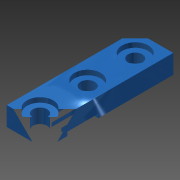
# Autodesk Inventor part: XCarriageBeltClamp
Saved by Autodesk Inventor 2015 (Build 190159000, 159)
## iProperties
Created: 2014-08-22
Part Number: XCarriageBeltClamp
Material: ABS Plastic
Document SubType Name: Modeling
Designer: t_clevj
Density: 1.06 g/cm^3
Appearance: Cyan
Author: t_clevj
Autodesk Inventor part; units mm, degrees
ref_plane "YZ Plane" through (0, 0, 0) normal (1, 0, 0) x (0, 1, 0)
ref_plane "XZ Plane" through (0, 0, 0) normal (0, 1, 0) x (-1, 0, 0)
ref_plane "XY Plane" through (0, 0, 0) normal (0, 0, 1) x (1, 0, 0)
sketch "Sketch1" plane through (0, 0, 0) normal (0, 0, 1) x (1, 0, 0)
  line L0 (0, 0) -> (8, 0)
  line L1 (8, 0) -> (8, 27)
  line L2 (8, 27) -> (0, 27)
  line L3 (0, 27) -> (0, 0)
  dimension "d0" = 27
  dimension "d1" = 8
  constraints: 8 end point, 2 parallel, 1 horizontal, 1 perpendicular
  measures "d0" distance of L2.end L0.start
  measures "d1" distance of L0.start L0.end
extrude "Extrusion1" add sketch "Sketch1" along normal blind 4
sketch "Sketch2" plane through (0, 0, 4) normal (0, 0, 1) x (1, 0, 0)
  line L0 (0, 0) -> (8, 0) projected
  line L1 (8, 0) -> (8, 27) projected
  point P0 (4, 23)
  point P1 (4, 13)
  point P2 (4, 3)
  dimension "d4" = 3
  dimension "d5" = 20
  dimension "d6" = 10
  dimension "d7" = 4
  constraints: 2 vertical alignment
  measures "d4" distance from line of L0 point (4, 3)
  measures "d5" distance of point (4, 23) point (4, 3)
  measures "d6" distance of point (4, 3) point (4, 13)
  measures "d7" distance from line of L1 point (4, 3)
hole "Hole1" at (4, 23, 4) at (4, 13, 4) at (4, 3, 4) direction (0, 0, -1) diameter 3 end up to face face through (2.6667, 18, 0) facing (0, 0, -1) counterbore diameter 5.5 counterbore depth 1
sketch "Sketch3" plane through (0, 0, 0) normal (0, 0, -1) x (-1, 0, 0)
  line L0 (-8, 0) -> (-8, 27) projected
  line L1 (-8, 21.25) -> (0, 21.25) construction
  line L2 (0, 27) -> (0, 0) construction
  line L3 (-8, 0) -> (-8, 27) construction
  line L4 (-8, 14.75) -> (0, 14.75) construction
  line L5 (-8, 21.25) -> (-6.7, 21.25)
  line L6 (-6.7, 21.25) -> (-6.7, 14.75)
  line L7 (-6.7, 14.75) -> (-8, 14.75)
  line L8 (-8, 14.75) -> (-8, 21.25)
  line L9 (-6, 21.25) -> (-4.7, 21.25)
  line L10 (-4.7, 21.25) -> (-4.7, 14.75)
  line L11 (-4.7, 14.75) -> (-6, 14.75)
  line L12 (-6, 14.75) -> (-6, 21.25)
  line L13 (-4, 21.25) -> (-2.7, 21.25)
  line L14 (-2.7, 21.25) -> (-2.7, 14.75)
  line L15 (-2.7, 14.75) -> (-4, 14.75)
  line L16 (-4, 14.75) -> (-4, 21.25)
  line L17 (-2, 21.25) -> (-0.7, 21.25)
  line L18 (-0.7, 21.25) -> (-0.7, 14.75)
  line L19 (-0.7, 14.75) -> (-2, 14.75)
  line L20 (-2, 14.75) -> (-2, 21.25)
  line L21 (-8, 21.25) -> (-8, 14.75)
  circle A0 centre (-4, 23) radius 1.5 projected
  dimension "d15" = 6.5
  dimension "d17" = 1.3
  dimension "d18" = 1.3
  dimension "d19" = 1.3
  dimension "d20" = 1.3
  dimension "d21" = 0.7
  dimension "d22" = 0.7
  dimension "d23" = 0.7
  dimension "d27" = 1.75
  constraints: 38 end point, 10 point on line, 9 parallel, 5 horizontal, 4 perpendicular, 1 midpoint, 1 vertical
  measures "d15" distance between parallel lines of L1 L4
  measures "d17" distance between parallel lines of L16 L14
  measures "d18" distance between parallel lines of L12 L10
  measures "d19" distance between parallel lines of L0 L6
  measures "d20" distance between parallel lines of L18 L20
  measures "d21" distance between parallel lines of L14 L20
  measures "d22" distance between parallel lines of L10 L16
  measures "d23" distance between parallel lines of L6 L12
  measures "d27" distance from line of A0.centre L1
extrude "Extrusion2" cut sketch "Sketch3" against normal blind 0.8 contours L0 L5 L6 L7 | L9 L10 L11 L12 | L13 L14 L15 L16 | L17 L18 L19 L20
body "Solid1"
